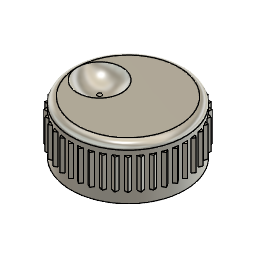
USB_Knob_Mag_screw v3 (Autodesk Fusion 360 design; units mm, degrees)
Autodesk Fusion 360 part; units mm, degrees
sketch "Sketch1" plane through (0, 0, 0) normal (0, 1, 0) x (1, 0, 0)
  circle A0 centre (0, 0) radius 17.95
  line L0 (0, 17.95) -> (0, 18.75)
  line L1 (0, 18.75) -> (0.8485, 17.9015)
  line L2 (0, 18.75) -> (1.2, 18.75) construction
  line L3 (0, 18.75) -> (-0.8485, 17.9015)
  line L4 (-2.9331, 18.5192) -> (-1.9623, 17.8138)
  line L5 (-2.9331, 18.5192) -> (-3.6385, 17.5483)
  line L6 (-5.7941, 17.8323) -> (-4.7249, 17.2875)
  line L7 (-5.7941, 17.8323) -> (-6.3389, 16.7631)
  line L8 (-8.5123, 16.7064) -> (-7.3711, 16.3356)
  line L9 (-8.5123, 16.7064) -> (-8.8831, 15.5651)
  line L10 (-11.021, 15.1691) -> (-9.8357, 14.9813)
  line L11 (-11.021, 15.1691) -> (-11.2087, 13.9838)
  line L12 (-13.2583, 13.2583) -> (-12.0583, 13.2583)
  line L13 (-13.2583, 13.2583) -> (-13.2583, 12.0583)
  line L14 (-15.1691, 11.021) -> (-13.9838, 11.2087)
  line L15 (-15.1691, 11.021) -> (-14.9813, 9.8357)
  line L16 (-16.7064, 8.5123) -> (-15.5651, 8.8831)
  line L17 (-16.7064, 8.5123) -> (-16.3356, 7.3711)
  line L18 (-17.8323, 5.7941) -> (-16.7631, 6.3389)
  line L19 (-17.8323, 5.7941) -> (-17.2875, 4.7249)
  line L20 (-18.5192, 2.9331) -> (-17.5483, 3.6385)
  line L21 (-18.5192, 2.9331) -> (-17.8138, 1.9623)
  line L22 (-18.75, 0) -> (-17.9015, 0.8485)
  line L23 (-18.75, 0) -> (-17.9015, -0.8485)
  line L24 (-18.5192, -2.9331) -> (-17.8138, -1.9623)
  line L25 (-18.5192, -2.9331) -> (-17.5483, -3.6385)
  line L26 (-17.8323, -5.7941) -> (-17.2875, -4.7249)
  line L27 (-17.8323, -5.7941) -> (-16.7631, -6.3389)
  line L28 (-16.7064, -8.5123) -> (-16.3356, -7.3711)
  line L29 (-16.7064, -8.5123) -> (-15.5651, -8.8831)
  line L30 (-15.1691, -11.021) -> (-14.9813, -9.8357)
  line L31 (-15.1691, -11.021) -> (-13.9838, -11.2087)
  line L32 (-13.2583, -13.2583) -> (-13.2583, -12.0583)
  line L33 (-13.2583, -13.2583) -> (-12.0583, -13.2583)
  line L34 (-11.021, -15.1691) -> (-11.2087, -13.9838)
  line L35 (-11.021, -15.1691) -> (-9.8357, -14.9813)
  line L36 (-8.5123, -16.7064) -> (-8.8831, -15.5651)
  line L37 (-8.5123, -16.7064) -> (-7.3711, -16.3356)
  line L38 (-5.7941, -17.8323) -> (-6.3389, -16.7631)
  line L39 (-5.7941, -17.8323) -> (-4.7249, -17.2875)
  line L40 (-2.9331, -18.5192) -> (-3.6385, -17.5483)
  line L41 (-2.9331, -18.5192) -> (-1.9623, -17.8138)
  line L42 (0, -18.75) -> (-0.8485, -17.9015)
  line L43 (0, -18.75) -> (0.8485, -17.9015)
  line L44 (2.9331, -18.5192) -> (1.9623, -17.8138)
  line L45 (2.9331, -18.5192) -> (3.6385, -17.5483)
  line L46 (5.7941, -17.8323) -> (4.7249, -17.2875)
  line L47 (5.7941, -17.8323) -> (6.3389, -16.7631)
  line L48 (8.5123, -16.7064) -> (7.3711, -16.3356)
  line L49 (8.5123, -16.7064) -> (8.8831, -15.5651)
  line L50 (11.021, -15.1691) -> (9.8357, -14.9813)
  line L51 (11.021, -15.1691) -> (11.2087, -13.9838)
  line L52 (13.2583, -13.2583) -> (12.0583, -13.2583)
  line L53 (13.2583, -13.2583) -> (13.2583, -12.0583)
  line L54 (15.1691, -11.021) -> (13.9838, -11.2087)
  line L55 (15.1691, -11.021) -> (14.9813, -9.8357)
  line L56 (16.7064, -8.5123) -> (15.5651, -8.8831)
  line L57 (16.7064, -8.5123) -> (16.3356, -7.3711)
  line L58 (17.8323, -5.7941) -> (16.7631, -6.3389)
  line L59 (17.8323, -5.7941) -> (17.2875, -4.7249)
  line L60 (18.5192, -2.9331) -> (17.5483, -3.6385)
  line L61 (18.5192, -2.9331) -> (17.8138, -1.9623)
  line L62 (18.75, 0) -> (17.9015, -0.8485)
  line L63 (18.75, 0) -> (17.9015, 0.8485)
  line L64 (18.5192, 2.9331) -> (17.8138, 1.9623)
  line L65 (18.5192, 2.9331) -> (17.5483, 3.6385)
  line L66 (17.8323, 5.7941) -> (17.2875, 4.7249)
  line L67 (17.8323, 5.7941) -> (16.7631, 6.3389)
  line L68 (16.7064, 8.5123) -> (16.3356, 7.3711)
  line L69 (16.7064, 8.5123) -> (15.5651, 8.8831)
  line L70 (15.1691, 11.021) -> (14.9813, 9.8357)
  line L71 (15.1691, 11.021) -> (13.9838, 11.2087)
  line L72 (13.2583, 13.2583) -> (13.2583, 12.0583)
  line L73 (13.2583, 13.2583) -> (12.0583, 13.2583)
  line L74 (11.021, 15.1691) -> (11.2087, 13.9838)
  line L75 (11.021, 15.1691) -> (9.8357, 14.9813)
  line L76 (8.5123, 16.7064) -> (8.8831, 15.5651)
  line L77 (8.5123, 16.7064) -> (7.3711, 16.3356)
  line L78 (5.7941, 17.8323) -> (6.3389, 16.7631)
  line L79 (5.7941, 17.8323) -> (4.7249, 17.2875)
  line L80 (2.9331, 18.5192) -> (3.6385, 17.5483)
  line L81 (2.9331, 18.5192) -> (1.9623, 17.8138)
  circle A1 centre (0, 0) radius 15.95
  point P0 (-1.5, 0)
  dimension "d1" = 35.9
  dimension "d15" = 0.8
  dimension "d16" = 45
  dimension "d17" = 1.2
  dimension "d25" = -2
  constraint coincident A0.centre A1.centre
  constraint coincident A0 L0.start
  constraint vertical L0
  constraint horizontal L2
  constraint symmetric L1.start L0 L2.start
  constraint symmetric L0 L1.end L3.end
  measures "d1" diameter of A0
  measures "d15" distance of L0.start L0.end
  measures "d16" angle of L1 L2
  measures "d17" distance of L0.end L1.end
extrude "Extrude1" add sketch "Sketch1" along normal blind 20 contours A0 | A1
extrude "Extrude4" add sketch "Sketch1" 1 faces at (-8.3371, 0, 5.9003) along normal blind 20 contours A0 L62 L63 | A0 L64 L65 | A0 L60 L61 | A0 L66 L67 | A0 L58 L59 | A0 L68 L69 | A0 L56 L57 | A0 L70 L71 | A0 L54 L55 | A0 L72 L73 | A0 L52 L53 | A0 L74 L75 | A0 L50 L51 | A0 L76 L77 | A0 L48 L49 | A0 L78 L79 | A0 L46 L47 | A0 L80 L81 | A0 L44 L45 | A0 L0 L1 | A0 L42 L43 | A0 L0 L3 | A0 L40 L41 | A0 L4 L5 | A0 L38 L39 | A0 L6 L7 | A0 L36 L37 | A0 L8 L9 | A0 L34 L35 | A0 L10 L11 | A0 L32 L33 | A0 L12 L13 | A0 L30 L31 | A0 L14 L15 | A0 L28 L29 | A0 L16 L17 | A0 L26 L27 | A0 L18 L19 | A0 L24 L25 | A0 L20 L21 | A0 L22 L23
extrude "Extrude5" add sketch "Sketch1" against normal blind 10 contours A0
sketch "Sketch3" plane through (0, -10, 0) normal (0, -1, 0) x (1, 0, 0)
  circle A0 centre (0, 0) radius 15.95
  circle A1 centre (0, 0) radius 17.95
  circle A2 centre (0, 0) radius 20
  dimension "d28" = 40
  constraint coincident A0.centre A1.centre
  measures "d28" diameter of A2
extrude "Extrude6" cut sketch "Sketch3" against normal blind 10 contours A1
extrude "Extrude7" cut sketch "Sketch3" against normal blind 17 contours A2
sketch "Sketch4" plane through (0, 20, 0) normal (0, 1, 0) x (-1, 0, 0)
  line L0 (17.8386, 1.9965) -> (18.5192, 2.9331)
  line L1 (18.5192, 2.9331) -> (17.5825, 3.6137)
  line L2 (17.3067, 4.7625) -> (17.8323, 5.7941)
  line L3 (17.8323, 5.7941) -> (16.8007, 6.3197)
  line L4 (16.3486, 7.4112) -> (16.7064, 8.5123)
  line L5 (16.7064, 8.5123) -> (15.6053, 8.8701)
  line L6 (14.988, 9.8774) -> (15.1691, 11.021)
  line L7 (15.1691, 11.021) -> (14.0255, 11.2021)
  line L8 (13.2583, 12.1005) -> (13.2583, 13.2583)
  line L9 (13.2583, 13.2583) -> (12.1005, 13.2583)
  line L10 (11.2021, 14.0255) -> (11.021, 15.1691)
  line L11 (11.021, 15.1691) -> (9.8774, 14.988)
  line L12 (8.8701, 15.6053) -> (8.5123, 16.7064)
  line L13 (8.5123, 16.7064) -> (7.4112, 16.3486)
  line L14 (6.3197, 16.8007) -> (5.7941, 17.8323)
  line L15 (5.7941, 17.8323) -> (4.7625, 17.3067)
  line L16 (3.6137, 17.5825) -> (2.9331, 18.5192)
  line L17 (2.9331, 18.5192) -> (1.9965, 17.8386)
  line L18 (0.8187, 17.9313) -> (0, 18.75)
  line L19 (0, 18.75) -> (-0.8187, 17.9313)
  line L20 (-1.9965, 17.8386) -> (-2.9331, 18.5192)
  line L21 (-2.9331, 18.5192) -> (-3.6137, 17.5825)
  line L22 (-4.7625, 17.3067) -> (-5.7941, 17.8323)
  line L23 (-5.7941, 17.8323) -> (-6.3197, 16.8007)
  line L24 (-7.4112, 16.3486) -> (-8.5123, 16.7064)
  line L25 (-8.5123, 16.7064) -> (-8.8701, 15.6053)
  line L26 (-9.8774, 14.988) -> (-11.021, 15.1691)
  line L27 (-11.021, 15.1691) -> (-11.2021, 14.0255)
  line L28 (-12.1005, 13.2583) -> (-13.2583, 13.2583)
  line L29 (-13.2583, 13.2583) -> (-13.2583, 12.1005)
  line L30 (-14.0255, 11.2021) -> (-15.1691, 11.021)
  line L31 (-15.1691, 11.021) -> (-14.988, 9.8774)
  line L32 (-15.6053, 8.8701) -> (-16.7064, 8.5123)
  line L33 (-16.7064, 8.5123) -> (-16.3486, 7.4112)
  line L34 (-16.8007, 6.3197) -> (-17.8323, 5.7941)
  line L35 (-17.8323, 5.7941) -> (-17.3067, 4.7625)
  line L36 (-17.5825, 3.6137) -> (-18.5192, 2.9331)
  line L37 (-18.5192, 2.9331) -> (-17.8386, 1.9965)
  line L38 (-17.9313, 0.8187) -> (-18.75, 0)
  line L39 (-18.75, 0) -> (-17.9313, -0.8187)
  line L40 (-17.8386, -1.9965) -> (-18.5192, -2.9331)
  line L41 (-18.5192, -2.9331) -> (-17.5825, -3.6137)
  line L42 (-17.3067, -4.7625) -> (-17.8323, -5.7941)
  line L43 (-17.8323, -5.7941) -> (-16.8007, -6.3197)
  line L44 (-16.3486, -7.4112) -> (-16.7064, -8.5123)
  line L45 (-16.7064, -8.5123) -> (-15.6053, -8.8701)
  line L46 (-14.988, -9.8774) -> (-15.1691, -11.021)
  line L47 (-15.1691, -11.021) -> (-14.0255, -11.2021)
  line L48 (-13.2583, -12.1005) -> (-13.2583, -13.2583)
  line L49 (-13.2583, -13.2583) -> (-12.1005, -13.2583)
  line L50 (-11.2021, -14.0255) -> (-11.021, -15.1691)
  line L51 (-11.021, -15.1691) -> (-9.8774, -14.988)
  line L52 (-8.8701, -15.6053) -> (-8.5123, -16.7064)
  line L53 (-8.5123, -16.7064) -> (-7.4112, -16.3486)
  line L54 (-6.3197, -16.8007) -> (-5.7941, -17.8323)
  line L55 (-5.7941, -17.8323) -> (-4.7625, -17.3067)
  line L56 (-3.6137, -17.5825) -> (-2.9331, -18.5192)
  line L57 (-2.9331, -18.5192) -> (-1.9965, -17.8386)
  line L58 (-0.8187, -17.9313) -> (0, -18.75)
  line L59 (0, -18.75) -> (0.8187, -17.9313)
  line L60 (1.9965, -17.8386) -> (2.9331, -18.5192)
  line L61 (2.9331, -18.5192) -> (3.6137, -17.5825)
  line L62 (4.7625, -17.3067) -> (5.7941, -17.8323)
  line L63 (5.7941, -17.8323) -> (6.3197, -16.8007)
  line L64 (7.4112, -16.3486) -> (8.5123, -16.7064)
  line L65 (8.5123, -16.7064) -> (8.8701, -15.6053)
  line L66 (9.8774, -14.988) -> (11.021, -15.1691)
  line L67 (11.021, -15.1691) -> (11.2021, -14.0255)
  line L68 (12.1005, -13.2583) -> (13.2583, -13.2583)
  line L69 (13.2583, -13.2583) -> (13.2583, -12.1005)
  line L70 (14.0255, -11.2021) -> (15.1691, -11.021)
  line L71 (15.1691, -11.021) -> (14.988, -9.8774)
  line L72 (15.6053, -8.8701) -> (16.7064, -8.5123)
  line L73 (16.7064, -8.5123) -> (16.3486, -7.4112)
  line L74 (16.8007, -6.3197) -> (17.8323, -5.7941)
  line L75 (17.8323, -5.7941) -> (17.3067, -4.7625)
  line L76 (17.5825, -3.6137) -> (18.5192, -2.9331)
  line L77 (18.5192, -2.9331) -> (17.8386, -1.9965)
  line L78 (17.9313, -0.8187) -> (18.75, 0)
  line L79 (18.75, 0) -> (17.9313, 0.8187)
  circle A0 centre (0, 0) radius 17.95
  circle A1 centre (0, 0) radius 15.95
  circle A2 centre (8.95, 0.0036) radius 7
  arc A3 (17.9313, 0.8187) -> (17.8386, 1.9965) centre (0, 0) ccw
  arc A4 (17.5825, 3.6137) -> (17.3067, 4.7625) centre (0, 0) ccw
  arc A5 (16.8007, 6.3197) -> (16.3486, 7.4112) centre (0, 0) ccw
  arc A6 (15.6053, 8.8701) -> (14.988, 9.8774) centre (0, 0) ccw
  arc A7 (14.0255, 11.2021) -> (13.2583, 12.1005) centre (0, 0) ccw
  arc A8 (12.1005, 13.2583) -> (11.2021, 14.0255) centre (0, 0) ccw
  arc A9 (9.8774, 14.988) -> (8.8701, 15.6053) centre (0, 0) ccw
  arc A10 (7.4112, 16.3486) -> (6.3197, 16.8007) centre (0, 0) ccw
  arc A11 (4.7625, 17.3067) -> (3.6137, 17.5825) centre (0, 0) ccw
  arc A12 (1.9965, 17.8386) -> (0.8187, 17.9313) centre (0, 0) ccw
  arc A13 (-0.8187, 17.9313) -> (-1.9965, 17.8386) centre (0, 0) ccw
  arc A14 (-3.6137, 17.5825) -> (-4.7625, 17.3067) centre (0, 0) ccw
  arc A15 (-6.3197, 16.8007) -> (-7.4112, 16.3486) centre (0, 0) ccw
  arc A16 (-8.8701, 15.6053) -> (-9.8774, 14.988) centre (0, 0) ccw
  arc A17 (-11.2021, 14.0255) -> (-12.1005, 13.2583) centre (0, 0) ccw
  arc A18 (-13.2583, 12.1005) -> (-14.0255, 11.2021) centre (0, 0) ccw
  arc A19 (-14.988, 9.8774) -> (-15.6053, 8.8701) centre (0, 0) ccw
  arc A20 (-16.3486, 7.4112) -> (-16.8007, 6.3197) centre (0, 0) ccw
  arc A21 (-17.3067, 4.7625) -> (-17.5825, 3.6137) centre (0, 0) ccw
  arc A22 (-17.8386, 1.9965) -> (-17.9313, 0.8187) centre (0, 0) ccw
  arc A23 (-17.9313, -0.8187) -> (-17.8386, -1.9965) centre (0, 0) ccw
  arc A24 (-17.5825, -3.6137) -> (-17.3067, -4.7625) centre (0, 0) ccw
  arc A25 (-16.8007, -6.3197) -> (-16.3486, -7.4112) centre (0, 0) ccw
  arc A26 (-15.6053, -8.8701) -> (-14.988, -9.8774) centre (0, 0) ccw
  arc A27 (-14.0255, -11.2021) -> (-13.2583, -12.1005) centre (0, 0) ccw
  arc A28 (-12.1005, -13.2583) -> (-11.2021, -14.0255) centre (0, 0) ccw
  arc A29 (-9.8774, -14.988) -> (-8.8701, -15.6053) centre (0, 0) ccw
  arc A30 (-7.4112, -16.3486) -> (-6.3197, -16.8007) centre (0, 0) ccw
  arc A31 (-4.7625, -17.3067) -> (-3.6137, -17.5825) centre (0, 0) ccw
  arc A32 (-1.9965, -17.8386) -> (-0.8187, -17.9313) centre (0, 0) ccw
  arc A33 (0.8187, -17.9313) -> (1.9965, -17.8386) centre (0, 0) ccw
  arc A34 (3.6137, -17.5825) -> (4.7625, -17.3067) centre (0, 0) ccw
  arc A35 (6.3197, -16.8007) -> (7.4112, -16.3486) centre (0, 0) ccw
  arc A36 (8.8701, -15.6053) -> (9.8774, -14.988) centre (0, 0) ccw
  arc A37 (11.2021, -14.0255) -> (12.1005, -13.2583) centre (0, 0) ccw
  arc A38 (13.2583, -12.1005) -> (14.0255, -11.2021) centre (0, 0) ccw
  arc A39 (14.988, -9.8774) -> (15.6053, -8.8701) centre (0, 0) ccw
  arc A40 (16.3486, -7.4112) -> (16.8007, -6.3197) centre (0, 0) ccw
  arc A41 (17.3067, -4.7625) -> (17.5825, -3.6137) centre (0, 0) ccw
  arc A42 (17.8386, -1.9965) -> (17.9313, -0.8187) centre (0, 0) ccw
  dimension "d33" = 35.9
  dimension "d34" = -2
  dimension "d54" = 14
  measures "d33" diameter of A0
  measures "d54" diameter of A2
ref_plane "WorkPlane1" through (0, 30, 0) normal (0, 1, 0) x (-1, 0, 0)
sketch "Sketch6" plane through (0, 30, 0) normal (0, 1, 0) x (1, 0, 0)
  circle A0 centre (0, 0) radius 20
  circle A1 centre (0, 0) radius 17.95
  dimension "d45" = 40
  dimension "d46" = 35.9
  constraint coincident A0.centre A1.centre
  measures "d45" diameter of A0
  measures "d46" diameter of A1
extrude "Extrude11" cut sketch "Sketch6" against normal blind 13.5
fillet "Fillet2" radius 2 1 edges at (-16.7353, 20, 6.491)
extrude "Extrude13" cut sketch "Sketch4" against normal blind 4 contours A2
fillet "Fillet3" radius 7 1 edges at (-2.4237, 16, 2.5349)
sketch "Sketch7" plane through (0, 0, 0) normal (0, 1, 0) x (1, 0, 0)
  circle A0 centre (0, 0) radius 17.95
  dimension "d59" = 35.9
  constraint coincident A0.centre origin
  measures "d59" diameter of A0
extrude "Extrude14" cut sketch "Sketch7" along normal blind 3.4
extrude "Extrude15" cut sketch "Sketch1" along normal blind 15 contours A1
thread "Thread2" "ISO Metric profile 32.0 M32x2 6H" major diameter 32.2565 minor diameter 30.0224 pitch 2 angle 60 modelled right hand crest width 0.5434 on face at (15.8707, 7.2667, -1.5881) crest through (15.0112, 3.9, 0)
